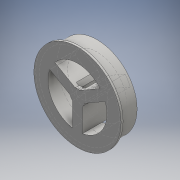
# Autodesk Inventor part: wheelPixi1
Saved by Autodesk Inventor 2016 (Build 200138000, 138)
## iProperties
Created: 2016-10-03
Part Number: wheelPixi1
Material: Generic
Document SubType Name: Modeling
Designer: skalp2
Density: 1 g/cm^3
Appearance: Default
Author: skalp2
Autodesk Inventor part; units mm, degrees
ref_plane "YZ Plane" through (0, 0, 0) normal (1, 0, 0) x (0, 1, 0)
ref_plane "XZ Plane" through (0, 0, 0) normal (0, 1, 0) x (-1, 0, 0)
ref_plane "XY Plane" through (0, 0, 0) normal (0, 0, 1) x (1, 0, 0)
sketch "Sketch1" plane through (0, 0, 0) normal (0, 1, 0) x (-1, 0, 0)
  circle A0 centre (0, 0) radius 11.75
  dimension "d0" = 23.5
  constraints: 1 centre point, 1 coincident
  measures "d0" diameter of A0
extrude "Extrusion1" add sketch "Sketch1" along normal blind 2.2
sketch "Sketch2" plane through (0, 0, 0) normal (0, -1, 0) x (1, 0, 0)
  circle A0 centre (0, 0) radius 16
  dimension "d3" = 32
  constraints: 1 centre point, 1 coincident
  measures "d3" diameter of A0
extrude "Extrusion2" add sketch "Sketch2" along normal blind 7
sketch "Sketch3" plane through (0, 2.2, 0) normal (0, 1, 0) x (1, 0, 0)
  arc A0 (-1.425, 1.2718) -> (1.425, 1.2718) centre (0, 0) ccw
  line L0 (-1.425, 1.2718) -> (1.425, 1.2718)
  dimension "d6" = 3.82
  dimension "d7" = 2.85
  constraints: 2 end point, 2 point on circle, 1 centre point, 1 coincident, 1 horizontal
  measures "d6" diameter of A0
  measures "d7" distance of L0.start L0.end
extrude "Extrusion3" cut sketch "Sketch3" against normal blind 8.5
sketch "Sketch6" plane through (0, -7, 0) normal (0, -1, 0) x (1, 0, 0)
  circle A0 centre (0, 0) radius 17.4
  circle A1 centre (0, 0) radius 16 projected
  dimension "d16" = 1.4
  constraints: 1 centre point, 1 coincident
  measures "d16" radial gap between concentric circles of A1 A0
extrude "Extrusion6" add sketch "Sketch6" along normal blind 0.8 contours A0 | A1
sketch "Sketch7" plane through (0, 2.2, 0) normal (0, 1, 0) x (1, 0, 0)
  circle A0 centre (0, 0) radius 11.75 projected
  line L0 (-1.425, 1.2718) -> (1.425, 1.2718) projected
  arc A1 (-1.425, 1.2718) -> (1.425, 1.2718) centre (0, 0) ccw projected
  circle A2 centre (0, 0) radius 11.75 projected
  line L1 (-2, 11.5785) -> (-2, 2.1889)
  line L2 (2, 2.1889) -> (2, 11.5785)
  line L3 (1.8733, 0.3725) -> (1.9126, 0.3725)
  line L4 (0, 0) -> (0, 15.765) construction
  line L5 (-2.8956, 0.6376) -> (-11.0273, -4.0572)
  line L6 (-9.0273, -7.5213) -> (-0.8956, -2.8265)
  line L7 (0.8956, -2.8265) -> (9.0273, -7.5213)
  line L8 (11.0273, -4.0572) -> (2.8956, 0.6376)
  line L9 (-1.525, 1.2942) -> (-1.525, 15.9272) projected
  arc A3 (11.0273, -4.0572) -> (2, 11.5785) centre (0, 0) ccw
  arc A4 (-2, 11.5785) -> (-11.0273, -4.0572) centre (0, 0) ccw
  arc A5 (-9.0273, -7.5213) -> (9.0273, -7.5213) centre (0, 0) ccw
  arc A6 (2.8956, 0.6376) -> (2, 2.1889) centre (0, 0) ccw
  arc A7 (-1.425, 1.2718) -> (1.425, 1.2718) centre (0, 0) ccw projected
  line L10 (1.965, -3.4439) -> (0, 0)
  line L11 (0, 0) -> (-1.965, -3.4439)
  arc A8 (1.4757, -2.5863) -> (-1.525, -2.5576) centre (0, 0) ccw
  arc A9 (-2, 2.1889) -> (-2.8956, 0.6376) centre (0, 0) ccw
  arc A10 (2.8956, 0.6376) -> (2, 2.1889) centre (0, 0) ccw
  arc A11 (1.4757, -2.5863) -> (-1.525, -2.5576) centre (0, 0) ccw
  dimension "d20" = 4
  dimension "d23" = 360
  constraints: 20 end point, 18 point on circle, 8 centre point, 4 point on line, 3 coincident, 1 parallel, 1 vertical, 23 other
  measures "d20" distance between parallel lines of L1 L2
extrude "Extrusion7" cut sketch "Sketch7" against normal blind 10 contours A0 L8 A8 L2 | A0 L6 L11 A1 L10 L7 | L1 A8 L5 A0 | A1 L11 L10
sketch "Sketch8" plane through (0, -7.8, 0) normal (0, -1, 0) x (1, 0, 0)
  arc A0 (2, -2.1889) -> (2.8956, -0.6376) centre (0, 0) ccw projected
  line L0 (0, 0) -> (-1.965, 3.4439) projected
  line L1 (-1.965, 3.4439) -> (-9.0273, 7.5213) projected
  line L2 (-1.965, 3.4439) -> (-0.8956, 2.8265)
  line L3 (0.8956, 2.8265) -> (1.965, 3.4439)
  line L4 (0.9466, 1.659) -> (1.965, 3.4439) projected
  line L5 (1.965, 3.4439) -> (1.4558, 2.5514)
  line L6 (-1.965, 3.4439) -> (-1.4694, 2.5753)
  arc A1 (-1.4694, 2.5753) -> (1.4694, 2.5753) centre (0, 0) ccw
  arc A2 (0.8956, 2.8265) -> (-0.8956, 2.8265) centre (0, 0) ccw
  constraints: 8 end point, 4 point on circle, 2 centre point, 2 point on line, 1 coincident, 1 collinear, 1 midpoint
extrude "Extrusion8" add sketch "Sketch8" against normal blind 1.5
body "Solid1"
